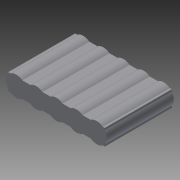
# Autodesk Inventor part: batterie_6v
Saved by Autodesk Inventor 2014 SP1 (Build 180222100, 222)
## iProperties
Created: 2015-02-02
Part Number: batterie_6v
Material: Générique
Document SubType Name: Modeling
Designer: astralien3000
Density: 1 g/cm^3
Appearance: Par défaut
Author: astralien3000
Autodesk Inventor part; units mm, degrees
ref_plane "YZ Plane" through (0, 0, 0) normal (1, 0, 0) x (0, 1, 0)
ref_plane "XZ Plane" through (0, 0, 0) normal (0, 1, 0) x (-1, 0, 0)
ref_plane "XY Plane" through (0, 0, 0) normal (0, 0, 1) x (1, 0, 0)
sketch "Esquisse1" plane through (0, 0, 0) normal (0, 1, 0) x (-1, 0, 0)
  circle A0 centre (-30, 0) radius 7.5
  circle A1 centre (30, 0) radius 7.5
  circle A2 centre (15, 0) radius 7.5
  circle A3 centre (0, 0) radius 7.5
  circle A4 centre (-15, 0) radius 7.5
  line L0 (0, 0) -> (-28.9231, 0) construction
  line L1 (-36, 6) -> (36, 6)
  line L2 (36, 6) -> (36, -6)
  line L3 (36, -6) -> (-36, -6)
  line L4 (-36, -6) -> (-36, 6)
  dimension "d0" = 15
  dimension "d1" = 15
  dimension "d2" = 15
  dimension "d3" = 15
  dimension "d4" = 15
  dimension "d7" = 12
  dimension "d8" = 6
  dimension "d9" = 72
  dimension "d10" = 36
  constraints: 10 end point, 5 centre point, 4 equal radius, 4 point on line, 2 horizontal, 2 parallel, 1 coincident, 1 perpendicular
  measures "d0" diameter of A4
  measures "d1" diameter of A3
  measures "d2" diameter of A2
  measures "d3" diameter of A1
  measures "d4" diameter of A0
  measures "d7" distance between parallel lines of L3 L1
  measures "d8" distance between parallel lines of L0 L3
  measures "d9" distance of L1.start L1.end
  measures "d10" distance from line of L0.start L2
extrude "Extrusion1" add sketch "Esquisse1" along normal blind 50
equation "\"d1\" = d0"
equation "\"d2\" = d0"
equation "\"d3\" = d0"
equation "\"d4\" = d0"
equation "\"d8\" = 0.5 * d7"
equation "\"d10\" = 0.5 * d9"
